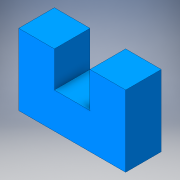
# Autodesk Inventor part: IED7_Sun_PuzzleCubeBlue
Saved by Autodesk Inventor 2016 (Build 200138000, 138)
## iProperties
Created: 2017-09-27
Part Number: IED7_Sun_PuzzleCubeBlue
Material: Generic
Document SubType Name: Sheet Metal
Designer: sun01147
Density: 1 g/cm^3
Sheet Metal Rule: Default
Appearance: Default
Author: sun01147
Autodesk Inventor part; units mm, degrees
ref_plane "YZ Plane" through (0, 0, 0) normal (1, 0, 0) x (0, 1, 0)
ref_plane "XZ Plane" through (0, 0, 0) normal (0, 1, 0) x (-1, 0, 0)
ref_plane "XY Plane" through (0, 0, 0) normal (0, 0, 1) x (1, 0, 0)
sketch "Sketch1" plane through (0, 0, 0) normal (0, 0, 1) x (1, 0, 0)
  point P0 (0, 0)
sketch "Sketch2" plane through (0, 0, 0) normal (0, 0, 1) x (1, 0, 0)
  line L0 (0, 38.1) -> (0, 0)
  line L1 (0, 0) -> (57.15, 0)
  line L2 (57.15, 0) -> (57.15, 38.1)
  line L3 (0, 38.1) -> (19.05, 38.1)
  line L4 (19.05, 38.1) -> (19.05, 19.05)
  line L5 (19.05, 19.05) -> (38.1, 19.05)
  line L6 (38.1, 19.05) -> (38.1, 38.1)
  line L7 (38.1, 38.1) -> (57.15, 38.1)
  dimension "d0" = 38.1
  dimension "d1" = 57.15
  dimension "d2" = 38.1
  dimension "d3" = 19.05
  dimension "d4" = 19.05
  dimension "d5" = 19.05
  constraints: 16 end point, 4 vertical, 3 horizontal, 1 perpendicular
  measures "d0" distance of L0.start L0.end
  measures "d1" distance of L0.end L1.end
  measures "d2" distance of L1.end L2.end
  measures "d3" distance of L0.start L3.end
  measures "d4" distance of L3.end L4.end
  measures "d5" distance of L4.end L5.end
extrude "Extrusion1" add sketch "Sketch2" along normal blind 19.05
equation "\"d0\" = 2 * cube"
equation "\"d1\" = 3 * cube"
equation "\"d2\" = 2 * cube"
equation "\"d3\" = cube"
equation "\"d4\" = cube"
equation "\"d5\" = cube"
equation "\"d6\" = cube"
equation "\"BendRadius\" = Thickness"
equation "\"BendReliefWidth\" = Thickness"
equation "\"BendReliefDepth\" = 0.5 * Thickness"
equation "\"CornerReliefSize\" = 4 * Thickness"
equation "\"MinimumRemnant\" = 2 * Thickness"
equation "\"TransitionRadius\" = BendRadius"
equation "\"JacobiRadiusSize\" = BendRadius"
equation "\"GapSize\" = Thickness"
equation "\"cube\" = 19.05"
equation "\"Thickness\" = 3.048"
body "Solid1"
